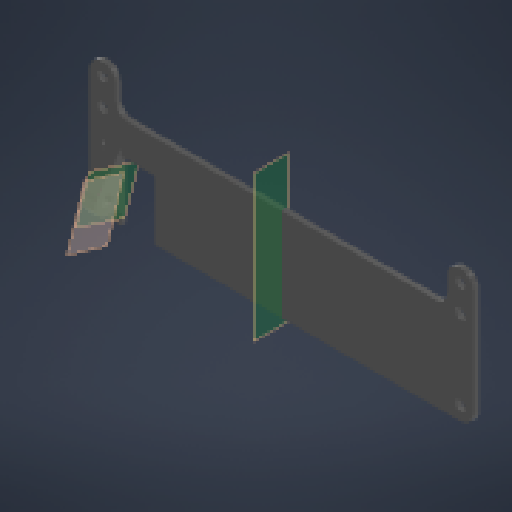
# Autodesk Inventor part: ramp
Saved by Autodesk Inventor 2025.2 (Build 292293000, 293)
## iProperties
Created: 2025-12-03
Part Number: ramp
Material: ABS Plastic
Document SubType Name: Modeling
Designer: cloudy
Mass: 23.006 g
Surface Area: 185.982 cm^2
Volume: 21.7037 cm^3
Density: 1.06 g/cm^3
Appearance: Smooth - Dark Gray
Author: cloudy
Autodesk Inventor part; units mm, degrees
ref_plane "YZ Plane" through (0, 0, 0) normal (1, 0, 0) x (0, 1, 0)
ref_plane "XZ Plane" through (0, 0, 0) normal (0, 1, 0) x (-1, 0, 0)
ref_plane "XY Plane" through (0, 0, 0) normal (0, 0, 1) x (1, 0, 0)
sketch "Sketch1" plane through (0, 0, 0) normal (0, 0, 1) x (1, 0, 0)
  circle A0 centre (0.7751, -44.45) radius 2.1844 projected
  circle A1 centre (0.7751, 6.35) radius 2.1844 projected
  circle A2 centre (0.7751, -6.35) radius 2.1844 projected
  circle A3 centre (172.2251, 6.35) radius 2.1844 projected
  circle A4 centre (172.2251, -6.35) radius 2.1844 projected
  circle A5 centre (172.2251, -44.45) radius 2.1844 projected
  arc A6 (-5.5749, -44.45) -> (0.7751, -50.8) centre (0.7751, -44.45) ccw
  arc A7 (7.1251, 6.35) -> (-5.5749, 6.35) centre (0.7751, 6.35) ccw
  arc A8 (178.5751, 6.35) -> (165.8751, 6.35) centre (172.2251, 6.35) ccw
  arc A9 (172.2251, -50.8) -> (178.5751, -44.45) centre (172.2251, -44.45) ccw
  line L0 (178.5751, 6.35) -> (178.5751, -44.45)
  line L1 (172.2251, -50.8) -> (0.7751, -50.8)
  line L2 (-5.5749, -44.45) -> (-5.5749, 6.35)
  line L3 (7.1251, -6.35) -> (165.8751, -6.35)
  line L4 (165.8751, -6.35) -> (165.8751, 6.7183)
  line L5 (7.1251, -6.35) -> (7.1251, 6.35)
  point P0 (0, 0)
  point P1 (223.8887, 136.6663)
  dimension "d0" = 12.7
  dimension "d2" = 44.45
  constraints: 14 end point, 8 point on circle, 8 tangent, 4 centre point, 4 coincident, 3 equal radius, 2 parallel, 1 point on line, 1 vertical, 1 other
  measures "d0" diameter of A9
  measures "d2" distance between parallel lines of L1 L3
extrude "Extrusion1" add sketch "Sketch1" along normal blind 2.54
fillet "Fillet1" radius 6.35 2 edges at (165.8751, -6.35, 1.27) (7.1251, -6.35, 1.27)
ref_plane "Work Plane2" through (9.8001, -34.7633, -2.5124) normal (-1, 0, 0) x (0, 0.3115065, 0.950244)
sketch "Sketch4" plane through (9.8001, -34.7633, -2.5124) normal (-1, 0, 0) x (0, 0.3115065, 0.950244)
  circle A0 centre (16.043, -8.0501) radius 2.1844
  line L0 (-0.63, -9.9873) -> (1.7836, -10.7786) projected
  line L1 (21.4074, -4.6521) -> (9.7994, 13.6734)
  line L2 (17.6081, 37.4938) -> (1.7836, -10.7786) projected
  line L3 (1.7836, -10.7786) -> (1.6106, -11.3063)
  circle A1 centre (16.043, -8.0501) radius 6.35
  line L4 (9.738, -7.2957) -> (3.5864, -5.2791)
  point P0 (13.2164, 32.251)
  dimension "d15" = 4.3688
  dimension "d51" = 12.7
  dimension "d52" = 12.7
  constraints: 6 end point, 3 point on line, 2 centre point, 2 point on circle, 1 coincident, 1 perpendicular, 1 tangent
  measures "d15" diameter of A0
  measures "d51" distance from line of L2 A0.centre
  measures "d52" diameter of A1
extrude "Extrusion3" add sketch "Sketch4" along normal blind 6.35
sketch "Sketch5" plane through (0, 0, 2.54) normal (0, 0, 1) x (1, 0, 0)
  arc A0 (178.5751, 6.35) -> (165.8751, 6.35) centre (172.2251, 6.35) ccw projected
  line L0 (165.8751, 6.35) -> (165.8751, 0) projected
  arc A1 (159.5251, -6.35) -> (165.8751, 0) centre (159.5251, 0) ccw projected
  line L1 (159.5251, -6.35) -> (13.4751, -6.35) projected
  arc A2 (7.1251, 0) -> (13.4751, -6.35) centre (13.4751, 0) ccw projected
  line L2 (7.1251, 0) -> (7.1251, 6.35) projected
  arc A3 (7.1251, 6.35) -> (-5.5749, 6.35) centre (0.7751, 6.35) ccw projected
  line L3 (-5.5749, 6.35) -> (-5.5749, -44.45) projected
  arc A4 (-5.5749, -44.45) -> (0.7751, -50.8) centre (0.7751, -44.45) ccw projected
  line L4 (0.7751, -50.8) -> (172.2251, -50.8) projected
  arc A5 (172.2251, -50.8) -> (178.5751, -44.45) centre (172.2251, -44.45) ccw projected
  line L5 (178.5751, -44.45) -> (178.5751, 6.35) projected
  circle A6 centre (0.7751, -6.35) radius 2.1844 projected
  circle A7 centre (172.2251, -6.35) radius 2.1844 projected
  circle A8 centre (172.2251, -44.45) radius 2.1844 projected
  circle A9 centre (172.2251, 6.35) radius 2.1844 projected
  circle A10 centre (0.7751, 6.35) radius 2.1844 projected
  circle A11 centre (0.7751, -44.45) radius 2.1844 projected
  line L6 (9.8001, -52.839) -> (25.6751, -52.839)
  line L7 (25.6751, -52.839) -> (25.6751, -22.225)
  line L8 (25.6751, -22.225) -> (9.8001, -22.225)
  line L9 (9.8001, -22.225) -> (9.8001, -52.839)
  point P0 (0, 0)
  dimension "d24" = 15.875
  constraints: 8 end point, 2 parallel, 1 horizontal, 1 perpendicular
  measures "d24" distance of L8.end L7.end
extrude "Extrusion4" cut sketch "Sketch5" against normal through all contours L7 L6 L9 L4 | L4 L9 L8 L7
chamfer "Chamfer1" distance 0.7937 angle 45 2 edges at (25.6751, -22.225, 1.27) (25.6751, -50.8, 1.27)
fillet "Fillet6" radius 3.175 2 edges at (6.6251, -38.6626, 9.0137) (6.6251, -38.6626, 2.54)
fillet "Fillet7" radius 3.175 2 edges at (3.4501, -40.2501, 2.54) (3.4501, -28.6901, 2.54)
sketch "Sketch6" plane through (0, 0, 2.54) normal (0, 0, 1) x (1, 0, 0)
  circle A0 centre (0.7751, -44.45) radius 2.1844 projected
  circle A1 centre (0.7751, -44.45) radius 4.7625
  point P0 (0, 0)
  point P1 (2.9595, -44.45)
  point P2 (2.9595, -44.45)
  dimension "d35" = 9.525
  constraints: 1 centre point, 1 coincident
  measures "d35" diameter of A1
extrude "Extrusion5" cut sketch "Sketch6" along normal blind 3.175 contours A0 | A1
ref_plane "Work Plane4" through (86.5001, -44.45, 0) normal (-1, 0, 0) x (0, 0, 1)
mirror "Mirror2" about plane through (86.5001, -44.45, 0) normal (-1, 0, 0) of "Extrusion5", "Fillet7", "Fillet6", "Extrusion4", "Chamfer1", "Extrusion3"
sketch "Sketch7" plane through (0, 0, 2.54) normal (0, 0, 1) x (1, 0, 0)
  line L0 (86.5001, -63.5) -> (86.5001, 25.4) projected
  line L1 (26.4689, -50.8) -> (146.5314, -50.8) projected
  circle A0 centre (45.2251, -44.45) radius 2.1844
  circle A1 centre (127.7751, -44.45) radius 2.1844
  point P0 (0, 0)
  dimension "d44" = 4.3688
  dimension "d45" = 41.275
  dimension "d46" = 41.275
  dimension "d47" = 6.35
  dimension "d48" = 6.35
  constraints: 2 centre point, 1 equal radius
  measures "d44" diameter of A0
  measures "d45" distance from line of A0.centre L0
  measures "d46" distance from line of A1.centre L0
  measures "d47" distance from line of L1 A0.centre
  measures "d48" distance from line of L1 A1.centre
extrude "Extrusion6" cut sketch "Sketch7" against normal through all
body "Solid1"
